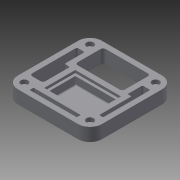
# Autodesk Inventor part: 14 pin shortest holder
Saved by Autodesk Inventor 2015 (Build 190159000, 159)
## iProperties
Created: 2014-12-11
Part Number: 14 pin shortest holder
Material: Generic
Document SubType Name: Modeling
Designer: Purple
Density: 1 g/cm^3
Appearance: Default
Author: Purple
Autodesk Inventor part; units mm, degrees
ref_plane "YZ Plane" through (0, 0, 0) normal (1, 0, 0) x (0, 1, 0)
ref_plane "XZ Plane" through (0, 0, 0) normal (0, 1, 0) x (-1, 0, 0)
sketch "Sketch1" plane through (0, 0, 0) normal (0, 1, 0) x (-1, 0, 0)
  line L0 (30, 30) -> (-30, 30)
  line L1 (-30, 30) -> (-30, -30)
  line L2 (-30, -30) -> (30, -30)
  line L3 (30, -30) -> (30, 30)
  line L4 (30, 30) -> (-30, -30) construction
  line L5 (-30, 30) -> (30, -30) construction
  point P0 (0, 0)
  dimension "d0" = 60
  dimension "d1" = 60
  constraints: 12 end point, 2 midpoint, 2 parallel, 1 horizontal, 1 perpendicular
  measures "d0" distance of L2.end L1.end
  measures "d1" distance of L0.end L1.end
extrude "Extrusion1" add sketch "Sketch1" along normal blind 10
fillet "Fillet1" radius 7 4 edges at (30, 5, 30) (30, 5, -30) (-30, 5, 30) (-30, 5, -30)
sketch "Sketch2" plane through (0, 10, 0) normal (0, 1, 0) x (1, 0, 0)
  line L0 (-30, 30) -> (30, 30)
  line L1 (30, 30) -> (30, -30)
  line L2 (30, -30) -> (-30, -30)
  line L3 (-30, -30) -> (-30, 30)
  line L4 (-30, 30) -> (30, -30) construction
  line L5 (30, 30) -> (-30, -30) construction
  line L6 (25, -25) -> (25, 25)
  line L7 (25, 25) -> (-25, 25)
  line L8 (-25, 25) -> (-25, -25)
  line L9 (-25, -25) -> (25, -25)
  circle A0 centre (25, -25) radius 2.75
  circle A1 centre (-25, -25) radius 2.75
  circle A2 centre (25, 25) radius 2.75
  circle A3 centre (-25, 25) radius 2.75
  point P0 (0, 0)
  dimension "d5" = 5
  dimension "d6" = 5.5
  dimension "d7" = 5.5
  dimension "d8" = 5.5
  dimension "d9" = 5.5
  constraints: 20 end point, 4 centre point, 4 coincident, 4 parallel, 2 midpoint, 2 perpendicular, 1 horizontal, 3 other
  measures "d5" distance between parallel lines of L1 L6
  measures "d6" diameter of A0
  measures "d7" diameter of A1
  measures "d8" diameter of A2
  measures "d9" diameter of A3
extrude "Extrusion2" cut sketch "Sketch2" against normal blind 3 contours L9 A0 L6 | L6 A0 L9 | A2 L7 L6 | L6 L7 A2 | A1 L8 L9 | L9 L8 A1 | A3 L8 L7 | L7 L8 A3
sketch "Sketch7" plane through (0, 10, 0) normal (0, 1, 0) x (1, 0, 0)
  line L0 (-23, 30) -> (23, 30)
  line L1 (30, 23) -> (30, -23)
  line L2 (23, -30) -> (-23, -30)
  line L3 (-30, -23) -> (-30, 23)
  line L4 (-30, 30) -> (30, -30) construction
  line L5 (30, 30) -> (-30, -30) construction
  arc A0 (-23, 30) -> (-30, 23) centre (-23, 23) ccw
  arc A1 (-30, -23) -> (-23, -30) centre (-23, -23) ccw
  arc A2 (23, -30) -> (30, -23) centre (23, -23) ccw
  arc A3 (30, 23) -> (23, 30) centre (23, 23) ccw
  line L6 (23, 32) -> (-23, 32)
  arc A4 (-23, 32) -> (-32, 23) centre (-23, 23) ccw
  line L7 (-32, 23) -> (-32, -23)
  arc A5 (-32, -23) -> (-23, -32) centre (-23, -23) ccw
  line L8 (-23, -32) -> (23, -32)
  arc A6 (23, -32) -> (32, -23) centre (23, -23) ccw
  line L9 (32, -23) -> (32, 23)
  arc A7 (32, 23) -> (23, 32) centre (23, 23) ccw
  point P0 (0, 0)
  dimension "d47" = 7
  dimension "d48" = 2
  constraints: 20 end point, 16 point on circle, 8 centre point, 8 point on line, 8 tangent, 4 parallel, 3 equal radius, 2 midpoint, 2 perpendicular, 1 horizontal, 7 other
  measures "d47" radius of A0
  measures "d48" distance between parallel lines of L0 L6
extrude "Extrusion6" add sketch "Sketch7" against normal blind 10
sketch "Sketch27" plane through (0, 10, 0) normal (0, 1, 0) x (1, 0, 0)
  line L0 (-25, 25) -> (25, 25)
  line L1 (25, 25) -> (25, -25)
  line L2 (25, -25) -> (-25, -25)
  line L3 (-25, -25) -> (-25, 25)
  line L4 (-25, 25) -> (25, -25) construction
  line L5 (25, 25) -> (-25, -25) construction
  line L6 (21, -21) -> (21, 21)
  line L7 (21, 21) -> (-21, 21)
  line L8 (-21, 21) -> (-21, -21)
  line L9 (-21, -21) -> (21, -21)
  line L10 (-13.8, -21) -> (-13.8, 2.6)
  line L11 (21, 2.6) -> (-13.8, 2.6)
  line L12 (19, 0.6) -> (-11.8, 0.6)
  line L13 (-11.8, 0.6) -> (-11.8, -20)
  line L14 (-19, -19) -> (-19, 19)
  line L15 (-19, 19) -> (19, 19)
  line L16 (20, 20) -> (20, 0.6)
  line L17 (-20, -20) -> (-20, 20)
  line L18 (-20, 20) -> (20, 20)
  line L19 (-13.8, -19) -> (-19, -19)
  line L20 (19, -20) -> (-11.8, -20)
  line L21 (-13.8, -20) -> (-20, -20)
  line L22 (19, 19) -> (19, 2.6)
  line L23 (19, 0.6) -> (19, -20)
  point P0 (0, 0)
  dimension "d266" = 50
  dimension "d267" = 50
  dimension "d268" = 4
  dimension "d269" = 34.8
  dimension "d270" = 23.6
  dimension "d271" = 2
  dimension "d273" = 1
  constraints: 48 end point, 10 parallel, 7 perpendicular, 5 point on line, 2 midpoint, 1 horizontal, 1 vertical, 5 other
  measures "d266" distance of L1.end L2.end
  measures "d267" distance of L0.end L1.end
  measures "d268" distance between parallel lines of L1 L6
  measures "d269" distance of L6.start L10.start
  measures "d270" distance of L6.start L11.start
  measures "d271" distance between parallel lines of L11 L12
  measures "d273" distance between parallel lines of L6 L16
extrude "Extrusion25" cut sketch "Sketch27" against normal blind 2 contours L9 L10 L11 L6
sketch "Sketch28" plane through (0, 10, 0) normal (0, 1, 0) x (1, 0, 0)
  line L0 (-11.8, 0.6) -> (19, 0.6)
  line L1 (19, 0.6) -> (19, -20)
  line L2 (19, -20) -> (-11.8, -20)
  line L3 (-11.8, -20) -> (-11.8, 0.6)
  point P0 (0, 0)
  constraints: 8 end point, 2 parallel, 1 horizontal, 1 perpendicular
extrude "Extrusion26" cut sketch "Sketch28" against normal blind 8
sketch "Sketch29" plane through (0, 10, 0) normal (0, 1, 0) x (1, 0, 0)
  line L0 (23, 32) -> (-23, 32) projected
  line L1 (-32, 23) -> (-32, -23) projected
  line L2 (32, -23) -> (32, 23) projected
  line L3 (-13.8, 2.6) -> (21, 2.6) projected
  line L4 (-18, 28) -> (18, 28)
  line L5 (18, 28) -> (18, 6.6)
  line L6 (18, 6.6) -> (-18, 6.6)
  line L7 (-18, 6.6) -> (-18, 28)
  line L8 (-23, -32) -> (23, -32) projected
  line L9 (21, 2.6) -> (21, -21) projected
  line L10 (28, 18) -> (22, 18)
  line L11 (22, 18) -> (22, 6.6)
  line L12 (22, 6.6) -> (25, 6.6)
  line L13 (28, 18) -> (28, -18)
  line L14 (28, -18) -> (25, -18)
  line L15 (25, -18) -> (25, 2.6)
  line L16 (25, 2.6) -> (25, 6.6)
  line L17 (21, -21) -> (-13.8, -21) projected
  line L18 (18, -28) -> (18, -25)
  line L19 (18, -25) -> (-18, -25)
  line L20 (-18, -25) -> (-18, -28)
  line L21 (-18, -28) -> (18, -28)
  line L22 (-13.8, -21) -> (-13.8, 2.6) projected
  line L23 (-28, -18) -> (-17.8, -18)
  line L24 (-17.8, -18) -> (-17.8, 2.6)
  line L25 (-17.8, 2.6) -> (-22, 2.6)
  line L26 (-22, 2.6) -> (-22, 6.6)
  line L27 (-28, 18) -> (-22, 18)
  line L28 (-22, 18) -> (-22, 6.6)
  line L29 (-28, 18) -> (-28, -18)
  point P0 (0, 0)
  dimension "d278" = 4
  dimension "d279" = 4
  dimension "d280" = 14
  dimension "d281" = 14
  dimension "d282" = 4
  dimension "d283" = 4
  dimension "d284" = 4
  dimension "d285" = 14
  dimension "d286" = 14
  dimension "d287" = 4
  dimension "d288" = 4
  dimension "d289" = 4
  dimension "d290" = 4
  dimension "d291" = 14
  dimension "d292" = 14
  dimension "d293" = 4
  dimension "d294" = 14
  dimension "d295" = 14
  dimension "d296" = 4
  dimension "d297" = 4
  dimension "d298" = 4
  dimension "d299" = 4
  dimension "d300" = 14
  dimension "d301" = 4
  constraints: 44 end point, 12 perpendicular, 2 horizontal, 2 vertical, 1 point on line
  measures "d278" distance from line of L0 L4.start
  measures "d279" distance from line of L0 L4.end
  measures "d280" distance from line of L1 L4.start
  measures "d281" distance from line of L4.end L2
  measures "d282" distance from line of L6.end L3
  measures "d283" distance from line of L2 L10.start
  measures "d284" distance from line of L2 L13.end
  measures "d285" distance from line of L0 L10.start
  measures "d286" distance from line of L13.end L8
  measures "d287" distance from line of L10.end L5
  measures "d288" distance from line of L9 L15.end
  measures "d289" distance from line of L8 L18.start
  measures "d290" distance from line of L8 L20.end
  measures "d291" distance from line of L2 L18.start
  measures "d292" distance from line of L1 L20.end
  measures "d293" distance from line of L17 L18.end
  measures "d294" distance from line of L8 L23.start
  measures "d295" distance from line of L8 L23.end
  measures "d296" distance from line of L22 L24.end
  measures "d297" distance from line of L7 L26.end
  measures "d298" distance from line of L1 L27.start
  measures "d299" distance from line of L22 L23.end
  measures "d300" distance from line of L0 L27.start
  measures "d301" distance from line of L1 L23.start
extrude "Extrusion27" cut sketch "Sketch29" against normal through all contours L4 L5 L6 L7 | L13 L14 L15 L16 L12 L11 L10 | L21 L20 L19 L18 | L29 L27 L28 L26 L25 L24 L23
ref_plane "Work Plane7" through (0, 5, 0) normal (0, 1, 0) x (1, 0, 0)
mirror "Mirror7" about plane through (0, 5, 0) normal (0, 1, 0) of "Extrusion2"
fillet "Fillet8" radius 2 6 edges at (18, 5, -28) (-18, 5, -28) (-18, 5, -6.6) (18, 5, -6.6) (-17.8, 5, 18) (-28, 5, 18)
fillet "Fillet8" radius 1 10 edges at (-28, 5, -18) (-22, 5, -18) (-22, 5, -2.6) (-17.8, 5, -2.6) (3.6, 2, -0.6) (19, 2, 9.7) (-11.8, 2, 9.7) (3.6, 2, 20) (28, 5, -18) (22, 5, -18)
fillet "Fillet8" radius 0.5 8 edges at (-18, 5, 28) (25, 5, 18) (25, 5, -6.6) (22, 5, -6.6) (28, 5, 18) (18, 5, 28) (18, 5, 25) (-18, 5, 25)
body "Solid1"
